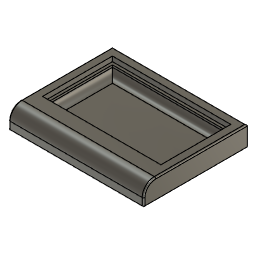
gaggia_tray (Autodesk Fusion 360 design; units mm, degrees)
Autodesk Fusion 360 part; units mm, degrees
sketch "Skizze1" plane through (0, 0, 0) normal (0, 0, 1) x (1, 0, 0)
  line L0 (0, 0) -> (195, 0)
  line L1 (195, 0) -> (195, 150)
  line L2 (195, 150) -> (0, 150)
  line L3 (0, 150) -> (0, 0)
  line L4 (0, 150) -> (42, 150) construction
  line L5 (42, 150) -> (42, 108) construction
  line L6 (42, 108) -> (0, 108) construction
  line L7 (0, 108) -> (0, 150) construction
  line L8 (195, 150) -> (153, 150) construction
  line L9 (153, 150) -> (153, 108) construction
  line L10 (153, 108) -> (195, 108) construction
  line L11 (195, 108) -> (195, 150) construction
  circle A0 centre (157.5, 112.5) radius 4.5
  circle A1 centre (37.5, 112.5) radius 4.5
  line L12 (0, 150) -> (12, 150) construction
  line L13 (12, 150) -> (12, 138) construction
  line L14 (12, 138) -> (0, 138) construction
  line L15 (0, 138) -> (0, 150) construction
  line L16 (12, 138) -> (183, 138)
  line L17 (183, 138) -> (183, 37)
  line L18 (183, 37) -> (12, 37)
  line L19 (12, 37) -> (12, 138)
  circle A2 centre (37.5, 112.5) radius 5.5
  circle A3 centre (157.5, 112.5) radius 5.5
  dimension "d1" = 195
  dimension "d2" = 150
  dimension "d3" = 42
  dimension "d4" = 42
  dimension "d5" = 42
  dimension "d6" = 42
  dimension "d7" = 4.5
  dimension "d8" = 4.5
  dimension "d9" = 12
  dimension "d10" = 12
  dimension "d11" = 171
  dimension "d12" = 101
  dimension "d41" = 1
  dimension "d42" = 1
  constraint horizontal L0
  constraint vertical L1
  constraint horizontal L2
  constraint vertical L3
  constraint coincident L0.start L3.end
  constraint horizontal L4
  constraint vertical L5
  constraint horizontal L6
  constraint vertical L7
  constraint horizontal L8
  constraint vertical L9
  constraint horizontal L10
  constraint vertical L11
  constraint tangent L10 A0
  constraint tangent L9 A0
  constraint tangent L6 A1
  constraint tangent L5 A1
  constraint horizontal L12
  constraint vertical L13
  constraint horizontal L14
  constraint vertical L15
  constraint horizontal L16
  constraint vertical L17
  constraint horizontal L18
  constraint vertical L19
  measures "d1" distance of L0.start L0.end
  measures "d2" distance of L0.start L2.end
  measures "d3" distance of L2.end L4.end
  measures "d4" distance of L2.end L6.end
  measures "d5" distance of L1.end L8.end
  measures "d6" distance of L1.end L10.end
  measures "d7" radius of A0
  measures "d8" radius of A1
  measures "d9" distance of L2.end L12.end
  measures "d10" distance of L2.end L14.end
  measures "d11" distance of L13.end L16.end
  measures "d12" distance of L13.end L18.end
extrude "Extrusion1" add sketch "Skizze1" along normal blind 30 contours L0 L1 L2 L3 | A0 | A1 | L16 L17 L18 L19 | A2 | A3 makes body 1
sketch "Skizze2" plane through (0, 0, 30) normal (0, 0, 1) x (-1, 0, 0)
  line L0 (0, -150) -> (0, 0)
  line L1 (0, 0) -> (-195, 0)
  line L2 (-195, 0) -> (-195, -150)
  line L3 (-195, -150) -> (0, -150)
  line L4 (0, -150) -> (-12, -150) construction
  line L5 (-12, -150) -> (-12, -138) construction
  line L6 (-12, -138) -> (0, -138) construction
  line L7 (0, -138) -> (0, -150) construction
  line L8 (-12, -138) -> (-183, -138)
  line L9 (-183, -138) -> (-183, -37)
  line L10 (-183, -37) -> (-12, -37)
  line L11 (-12, -37) -> (-12, -138)
  line L12 (-179, -41) -> (-16, -41)
  line L13 (-16, -41) -> (-16, -134)
  line L14 (-16, -134) -> (-179, -134)
  line L15 (-179, -134) -> (-179, -41)
  dimension "d15" = 12
  dimension "d16" = 12
  dimension "d17" = 171
  dimension "d18" = 101
  dimension "d19" = 4
  constraint horizontal L4
  constraint vertical L5
  constraint horizontal L6
  constraint vertical L7
  constraint coincident L0.start L3.end
  constraint horizontal L8
  constraint vertical L9
  constraint horizontal L10
  constraint vertical L11
  measures "d15" distance of L0.start L4.end
  measures "d16" distance of L0.start L6.end
  measures "d17" distance of L5.end L8.end
  measures "d18" distance of L5.end L10.end
extrude "Extrusion2" cut sketch "Skizze2" against normal blind 7 contours L8 L9 L10 L11 | L12 L13 L14 L15 bodies 1
extrude "Extrusion3" cut sketch "Skizze2" against normal blind 20 contours L12 L13 L14 L15 bodies 1
fillet "Abrundung1" radius 17.5 1 edges at (97.5, 0, 30) on bodies 1
fillet "Abrundung4" radius 10 4 edges at (97.5, 134, 10) (16, 87.5, 10) (179, 87.5, 10) (97.5, 41, 10) on bodies 1
fillet "Abrundung5" radius 2 7 edges at (97.5, 150, 30) (0, 83.75, 30) (0, 5.1256, 24.8744) (0, 0, 6.25) (195, 0, 6.25) (195, 5.1256, 24.8744) (195, 83.75, 30) on bodies 1
chamfer "Fase1" distance 2 angle 45 5 edges at (97.5, 0, 0) (194.4142, 0.5858, 0) (195, 76, 0) (0, 76, 0) (0.5858, 0.5858, 0) on bodies 1
extrude "Extrusion5" cut sketch "Skizze1" along normal blind 1 contours A0 | A1 | A2 | A3 bodies 1
extrude "Extrusion6" add sketch "Skizze1" along normal blind 2.5 separate body contours A0 | A1 makes body 2 at (33.0224, 112.0519, 1.6667) makes body 3 at (153.0224, 112.0519, 1.6667)
move_body "Verschieben1" bodies 3 2 to x (1, 0, 0) y (0, 1, 0) z (0, 0, 1) at (0, 0, -1.5)
